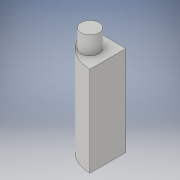
# Autodesk Inventor part: FanLegs
Saved by Autodesk Inventor 2019 (Build 230136000, 136)
## iProperties
Created: 2018-06-18
Part Number: FanLegs
Material: Ogólny
Document SubType Name: Modeling
Designer: Kamil
Density: 1 g/cm^3
Appearance: Domyślna
Author: Kamil
Autodesk Inventor part; units mm, degrees
ref_plane "YZ Plane" through (0, 0, 0) normal (1, 0, 0) x (0, 1, 0)
ref_plane "XZ Plane" through (0, 0, 0) normal (0, 1, 0) x (-1, 0, 0)
ref_plane "XY Plane" through (0, 0, 0) normal (0, 0, 1) x (1, 0, 0)
sketch "Szkic1" plane through (0, 0, 0) normal (0, 1, 0) x (-1, 0, 0)
  line L0 (-2, 2) -> (2, 2)
  line L1 (2, 2) -> (2, -2)
  line L2 (2, -2) -> (-2, -2)
  line L3 (-2, -2) -> (-2, 2)
  line L4 (-2, 2) -> (2, -2) construction
  line L5 (2, 2) -> (-2, -2) construction
  point P0 (0, 0)
  dimension "d0" = 4
  dimension "d1" = 4
  constraints: 12 end point, 2 midpoint, 2 parallel, 1 horizontal, 1 perpendicular
  measures "d0" distance of L1.end L2.end
  measures "d1" distance of L0.end L1.end
extrude "Wyciągnięcie proste1" add sketch "Szkic1" along normal blind 10
fillet "Zaokrąglenie1" radius 4 1 edges at (-2, 5, 2)
sketch "Szkic2" plane through (0, 10, 0) normal (0, 1, 0) x (1, 0, 0)
  circle A0 centre (0, 0) radius 1
  dimension "d5" = 2
  constraints: 1 centre point, 1 coincident
  measures "d5" diameter of A0
extrude "Wyciągnięcie proste2" add sketch "Szkic2" along normal blind 2
